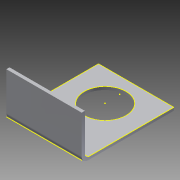
# Autodesk Inventor part: back support PG-71
Saved by Autodesk Inventor 2013 (Build 170138000, 138)
## iProperties
Created: 2013-02-02
Part Number: back support PG-71
Material: Aluminum 6061
Document SubType Name: Sheet Metal
Designer: aslane
Density: 1 g/cm^3
Sheet Metal Rule: Default
Author: aslane
Autodesk Inventor part; units mm, degrees
ref_plane "YZ Plane" through (0, 0, 0) normal (1, 0, 0) x (0, 1, 0)
ref_plane "XZ Plane" through (0, 0, 0) normal (0, 1, 0) x (-1, 0, 0)
ref_plane "XY Plane" through (0, 0, 0) normal (0, 0, 1) x (1, 0, 0)
sketch "Sketch1" plane through (0, 0, 0) normal (0, 1, 0) x (-1, 0, 0)
  line L0 (0, 0) -> (37.3126, 0)
  line L1 (37.3126, 0) -> (37.3126, 50.8)
  line L2 (37.3126, 50.8) -> (0, 50.8)
  line L3 (0, 50.8) -> (0, 0)
  line L4 (0, 0) -> (-38.1, 0)
  line L5 (-38.1, 0) -> (-38.1, 50.8)
  line L6 (-38.1, 50.8) -> (0, 50.8)
  line L7 (37.3126, 50.8) -> (37.3126, 76.2)
  line L8 (37.3126, 76.2) -> (0, 76.2)
  line L9 (0, 76.2) -> (-38.1, 76.2)
  line L10 (-38.1, 76.2) -> (-38.1, 50.8)
  line L11 (0, 76.2) -> (0, 50.8)
  dimension "d0" = 37.3126
  dimension "d1" = 50.8
  dimension "d2" = 38.1
  dimension "d3" = 25.4
  measures "d0" distance of L0.start L0.end
  measures "d1" distance of L0.end L1.end
  measures "d2" distance of L0.start L4.end
  measures "d3" distance of L1.end L7.end
extrude "Plate1" add sketch "Sketch1" along normal blind 3.175
sketch "Sketch2" plane through (38.1, 0, 73.025) normal (0, 0, 1) x (1, 0, 0)
  line L0 (-75.4126, 0) -> (0, 0)
  line L1 (0, 0) -> (0, 38.1)
  line L2 (0, 38.1) -> (-75.4126, 38.1)
  line L3 (-75.4126, 38.1) -> (-75.4126, 0)
  constraints: 6 end point, 1 horizontal, 1 perpendicular, 1 vertical
edge flange "Flange1" height 38.1 angle 90 thickness 3.175 bend radius 3.175 thickness toward (0, 0, 1) relief straight relief width 3.175 relief depth 1.5875 edges at (0.3937, 3.175, 76.2) wall of the first edge with corners at (-37.3126, 0, 73.025) (38.1, 0, 73.025) (38.1, 38.1, 73.025) (-37.3126, 38.1, 73.025)
bend "Bend1"
corner "Corner1"
sketch "Sketch3" plane through (0, 3.175, 0) normal (0, 1, 0) x (1, 0, 0)
  line L0 (-37.3126, 0) -> (38.1, 0)
  line L1 (-37.3126, -69.85) -> (-37.3126, 0)
  line L2 (-37.3126, 0) -> (-37.3126, 19.05)
  line L3 (-37.3126, 19.05) -> (38.1, 19.05)
  line L4 (38.1, 19.05) -> (38.1, 0)
  point P0 (0, 0)
  dimension "d15" = 19.05
  measures "d15" distance of L0.start L2.end
sheet face with bend "Face2" sketch "Sketch3" thickness 3.175 toward (0, -1, 0) bend radius 3.175 relief straight relief width 3.175 relief depth 1.5875
bend "Bend2"
sketch "Sketch4" plane through (-37.3126, 38.1, 76.2) normal (0, 1, 0) x (1, 0, 0)
  line L0 (0, 0) -> (75.4126, 0) projected
  line L1 (75.4126, 3.175) -> (75.4126, 0) projected
  line L2 (0, 3.175) -> (75.4126, 3.175) projected
  line L3 (0, 3.175) -> (0, 0) projected
  point P0 (37.3126, 76.2)
extrude "Extrusion1" add sketch "Sketch4" along normal blind 6.35
sketch "Sketch5" plane through (38.1, 3.175, -19.05) normal (0, 0, -1) x (-1, 0, 0)
  line L0 (0, -3.175) -> (75.4126, -3.175) projected
  line L1 (75.4126, 0) -> (75.4126, -3.175) projected
  line L2 (0, 0) -> (75.4126, 0) projected
  line L3 (0, 0) -> (0, -3.175) projected
  point P0 (38.1, -3.175)
extrude "Extrusion2" cut sketch "Sketch5" against normal blind 3.175
sketch "Sketch6" plane through (0, 3.175, 0) normal (0, 1, 0) x (1, 0, 0)
  line L0 (38.1, 15.875) -> (-37.3126, 15.875) projected
  line L1 (38.1, 15.875) -> (38.1, -69.85) projected
  line L2 (0.3937, 15.875) -> (0.3937, -15.1638)
  circle A0 centre (0.3937, -15.1638) radius 20.9169
  point P0 (0, 0)
  dimension "d25" = 31.0388
  dimension "d26" = 41.8338
  constraints: 2 end point, 1 centre point, 1 coincident, 1 midpoint, 1 parallel
  measures "d25" distance of L2.start L2.end
  measures "d26" diameter of A0
extrude "Cut1" cut sketch "Sketch6" against normal blind 3.175
sketch "Sketch7" plane through (0, 3.175, 0) normal (0, 1, 0) x (1, 0, 0)
  circle A0 centre (0.3937, -15.1638) radius 20.9169 projected
  line L0 (38.1, 15.875) -> (-37.3126, 15.875) projected
  line L1 (-37.3126, 15.875) -> (-37.3126, -69.85) projected
  line L2 (-37.3126, -69.85) -> (38.1, -69.85) projected
  line L3 (38.1, 15.875) -> (38.1, -69.85) projected
  line L4 (-37.3126, -76.2) -> (38.1, -76.2) projected
  point P0 (0, 0)
equation "\"d27\" = Thickness"
equation "\"d5\" = BendReliefWidth"
equation "\"d6\" = BendReliefDepth"
equation "\"d7\" = MinimumRemnant"
equation "\"d8\" = BendRadius"
equation "\"d11\" = BendRadius"
equation "\"d12\" = CornerReliefSize"
equation "\"d13\" = GapSize"
equation "\"d14\" = JacobiRadiusSize"
equation "\"d16\" = BendRadius"
equation "\"d17\" = BendReliefWidth"
equation "\"d19\" = MinimumRemnant"
equation "\"d18\" = BendReliefDepth"
equation "\"d20\" = BendRadius"
equation "\"BendRadius\" = Thickness"
equation "\"BendReliefWidth\" = Thickness"
equation "\"BendReliefDepth\" = 0.5 * Thickness"
equation "\"CornerReliefSize\" = 4 * Thickness"
equation "\"MinimumRemnant\" = 2 * Thickness"
equation "\"TransitionRadius\" = BendRadius"
equation "\"JacobiRadiusSize\" = BendRadius"
equation "\"GapSize\" = Thickness"
equation "\"d4\" = BendRadius"
equation "\"Thickness\" = 3.175"
body "Solid1"
